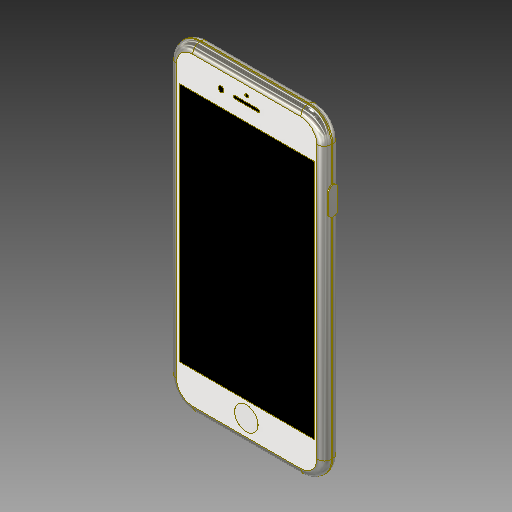
# Autodesk Inventor part: Iphone - Athena H
Saved by Autodesk Inventor 2019 (Build 230136000, 136)
## iProperties
Created: 2018-11-30
Part Number: Iphone - Athena H
Material: Generic
Document SubType Name: Modeling
Designer: mhs
Density: 1 g/cm^3
Appearance: Default
Author: mhs
Autodesk Inventor part; units mm, degrees
ref_plane "YZ Plane" through (0, 0, 0) normal (1, 0, 0) x (0, 1, 0)
ref_plane "XZ Plane" through (0, 0, 0) normal (0, 1, 0) x (-1, 0, 0)
ref_plane "XY Plane" through (0, 0, 0) normal (0, 0, 1) x (1, 0, 0)
sketch "Sketch1" plane through (0, 0, 0) normal (0, 0, 1) x (1, 0, 0)
  line L0 (10.16, 0) -> (56.896, 0)
  line L1 (67.056, 10.16) -> (67.056, 128.016)
  line L2 (56.896, 138.176) -> (10.16, 138.176)
  line L3 (0, 128.016) -> (0, 10.16)
  arc A0 (10.16, 138.176) -> (0, 128.016) centre (10.16, 128.016) ccw
  arc A1 (67.056, 128.016) -> (56.896, 138.176) centre (56.896, 128.016) ccw
  arc A2 (56.896, 0) -> (67.056, 10.16) centre (56.896, 10.16) ccw
  arc A3 (0, 10.16) -> (10.16, 0) centre (10.16, 10.16) ccw
  line L4 (4.318, 121.158) -> (62.738, 121.158)
  line L5 (62.738, 121.158) -> (62.738, 17.018)
  line L6 (62.738, 17.018) -> (4.318, 17.018)
  line L7 (4.318, 17.018) -> (4.318, 121.158)
  point P0 (0, 0)
  point P1 (67.056, 138.176)
  point P2 (67.056, 0)
  point P3 (0, 138.176)
  dimension "d0" = 67.056
  dimension "d1" = 138.176
  dimension "d2" = 10.16
  dimension "d3" = 58.42
  dimension "d4" = 104.14
  dimension "d5" = 17.018
  dimension "d6" = 4.318
  constraints: 16 end point, 8 point on circle, 8 point on line, 8 tangent, 4 centre point, 4 parallel, 3 equal radius, 2 horizontal, 2 perpendicular
  measures "d0" distance of point (67.056, 138.176) point (0, 138.176)
  measures "d1" distance of point (67.056, 0) point (67.056, 138.176)
  measures "d2" radius of A0
  measures "d3" distance of L4.start L4.end
  measures "d4" distance of L4.end L5.end
  measures "d5" distance between parallel lines of L0 L6
  measures "d6" distance between parallel lines of L3 L7
extrude "Extrusion1" add sketch "Sketch1" along normal blind 6.858 contours A3 L3 A0 L2 A1 L1 A2 L0 | L4 L5 L6 L7
fillet "Fillet1" radius 3.175 16 edges at (64.0802, 135.2002, 6.858) (33.528, 138.176, 6.858) (2.9758, 135.2002, 6.858) (0, 69.088, 6.858) (2.9758, 2.9758, 6.858) (33.528, 0, 6.858) (64.0802, 2.9758, 6.858) (67.056, 69.088, 6.858) (64.0802, 135.2002, 0) (33.528, 138.176, 0) (2.9758, 135.2002, 0) (0, 69.088, 0) (2.9758, 2.9758, 0) (33.528, 0, 0) (64.0802, 2.9758, 0) (67.056, 69.088, 0)
sketch "Sketch2" plane through (0, 0, 6.858) normal (0, 0, 1) x (1, 0, 0)
  line L0 (4.318, 121.158) -> (62.738, 121.158)
  line L1 (62.738, 121.158) -> (62.738, 17.018)
  line L2 (62.738, 17.018) -> (4.318, 17.018)
  line L3 (4.318, 17.018) -> (4.318, 121.158)
  line L4 (56.896, 138.176) -> (10.16, 138.176) projected
  line L5 (0, 128.016) -> (0, 10.16) projected
  point P0 (0, 0)
  dimension "d10" = 104.14
  dimension "d11" = 58.42
  dimension "d12" = 17.018
  dimension "d13" = 4.318
  constraints: 8 end point, 2 parallel, 1 horizontal, 1 perpendicular
  measures "d10" distance of L2.end L0.start
  measures "d11" distance of L0.start L0.end
  measures "d12" distance between parallel lines of L4 L0
  measures "d13" distance between parallel lines of L3 L5
extrude "Extrusion2" add sketch "Sketch2" along normal blind 0.0254
sketch "Sketch3" plane through (0, 0, 6.858) normal (0, 0, 1) x (1, 0, 0)
  circle A0 centre (33.401, 10.3132) radius 5.08
  line L0 (63.881, 128.016) -> (63.881, 10.16) projected
  point P0 (0, 0)
  dimension "d16" = 10.16
  dimension "d17" = 30.48
  constraints: 1 centre point
  measures "d16" diameter of A0
  measures "d17" distance from line of L0 A0.centre
extrude "Extrusion3" add sketch "Sketch3" along normal blind 0.0254
sketch "Sketch4" plane through (0, 0, 6.858) normal (0, 0, 1) x (1, 0, 0)
  line L0 (28.448, 128.016) -> (38.608, 128.016) construction
  line L1 (10.16, 135.001) -> (56.896, 135.001) projected
  line L2 (28.448, 127.381) -> (38.608, 127.381)
  line L3 (38.608, 128.651) -> (28.448, 128.651)
  arc A0 (28.448, 128.651) -> (28.448, 127.381) centre (28.448, 128.016) ccw
  arc A1 (38.608, 127.381) -> (38.608, 128.651) centre (38.608, 128.016) ccw
  circle A2 centre (22.479, 128.016) radius 1.27
  circle A3 centre (33.528, 131.1287) radius 0.762
  point P0 (0, 0)
  point P1 (33.528, 128.016)
  point P2 (33.528, 135.001)
  point P3 (33.528, 128.651)
  point P4 (63.881, 128.016)
  point P5 (39.243, 128.016)
  point P6 (3.175, 128.016)
  dimension "d20" = 1.27
  dimension "d21" = 10.16
  dimension "d22" = 2.54
  dimension "d23" = 4.064
  dimension "d24" = 1.524
  dimension "d25" = 2.4777
  constraints: 8 end point, 5 point on circle, 4 centre point, 4 tangent, 3 midpoint, 2 horizontal alignment, 2 parallel, 1 vertical alignment
  measures "d20" diameter of A1
  measures "d21" distance of L2.start L2.end
  measures "d22" diameter of A2
  measures "d24" diameter of A3
  measures "d25" distance from line of A3.centre L3
extrude "Extrusion4" cut sketch "Sketch4" against normal blind 0.0254
sketch "Sketch5" plane through (0, 0, 0) normal (0, 0, -1) x (-1, 0, 0)
  circle A0 centre (-52.7685, 127.0635) radius 3.175
  line L0 (-63.881, 10.16) -> (-63.881, 128.016) projected
  line L1 (-56.896, 135.001) -> (-10.16, 135.001) projected
  point P0 (0, 0)
  dimension "d28" = 6.35
  dimension "d29" = 11.1125
  dimension "d30" = 4.7625
  constraints: 1 centre point
  measures "d28" diameter of A0
  measures "d29" distance from line of A0.centre L0
  measures "d30" distance edge to line of A0 L1
extrude "Extrusion5" add sketch "Sketch5" along normal blind 1.27 draft -10
sketch "Sketch6" plane through (0, 0, 0) normal (0, 0, -1) x (-1, 0, 0)
  circle A0 centre (-46.4185, 127.0635) radius 0.5
  circle A1 centre (-40.0685, 127.0635) radius 2
  line L0 (-56.896, 135.001) -> (-10.16, 135.001) projected
  circle A2 centre (-52.7685, 127.0635) radius 2.9511 projected
  point P0 (0, 0)
  dimension "d33" = 1
  dimension "d34" = 4
  dimension "d35" = 7.9375
  dimension "d36" = 7.9375
  dimension "d37" = 6.35
  dimension "d38" = 6.35
  constraints: 2 centre point
  measures "d33" diameter of A0
  measures "d34" diameter of A1
  measures "d35" distance from line of L0 A1.centre
  measures "d36" distance from line of L0 A0.centre
  measures "d37" distance of A0.centre A2.centre
  measures "d38" distance of A0.centre A1.centre
extrude "Extrusion6" add sketch "Sketch6" along normal blind 0.0254 contours A0 | A1
sketch "Sketch7" plane through (67.056, 10.16, 3.175) normal (1, 0, 0) x (0, 0, -1)
  line L0 (-0.254, 100.856) -> (-0.254, 92.856) construction
  line L1 (0, 117.856) -> (0, 0) projected
  line L2 (-2.254, 100.856) -> (-2.254, 92.856)
  line L3 (1.746, 92.856) -> (1.746, 100.856)
  arc A0 (1.746, 100.856) -> (-2.254, 100.856) centre (-0.254, 100.856) ccw
  arc A1 (-2.254, 92.856) -> (1.746, 92.856) centre (-0.254, 92.856) ccw
  line L4 (0, 117.856) -> (-0.508, 117.856) projected
  line L5 (3.175, 117.856) -> (0, 117.856) projected
  point P0 (3.175, -10.16)
  point P1 (-0.254, 96.856)
  point P2 (-0.254, 117.856)
  dimension "d41" = 8
  dimension "d42" = 2
  dimension "d43" = 17
  constraints: 8 end point, 4 point on circle, 4 tangent, 2 centre point, 2 midpoint, 2 parallel, 1 vertical alignment
  measures "d41" distance of L2.start L2.end
  measures "d42" radius of A0
  measures "d43" distance from line of L0.start L5
extrude "Extrusion7" add sketch "Sketch7" along normal blind 0.508
sketch "Sketch8" plane through (0, 10.16, 3.175) normal (-1, 0, 0) x (0, 0, 1)
  line L0 (0.254, 113.856) -> (0.254, 109.856) construction
  line L1 (0, 117.856) -> (0, 102.8398) projected
  line L2 (-1.246, 113.856) -> (-1.246, 109.856)
  line L3 (1.754, 109.856) -> (1.754, 113.856)
  arc A0 (1.754, 113.856) -> (-1.246, 113.856) centre (0.254, 113.856) ccw
  arc A1 (-1.246, 109.856) -> (1.754, 109.856) centre (0.254, 109.856) ccw
  line L4 (0.254, 101.856) -> (0.254, 81.856) construction
  line L5 (-1.746, 101.856) -> (-1.746, 81.856)
  line L6 (2.254, 81.856) -> (2.254, 101.856)
  arc A2 (2.254, 101.856) -> (-1.746, 101.856) centre (0.254, 101.856) ccw
  arc A3 (-1.746, 81.856) -> (2.254, 81.856) centre (0.254, 81.856) ccw
  line L7 (0, 117.856) -> (0.508, 117.856) projected
  point P0 (-3.175, -10.16)
  point P1 (0.254, 111.856)
  point P2 (0.254, 91.856)
  point P3 (0.254, 117.856)
  point P4 (0.254, 117.856)
  dimension "d46" = 1.5
  dimension "d47" = 2
  dimension "d48" = 4
  dimension "d49" = 4
  dimension "d50" = 8
  dimension "d51" = 20
  constraints: 16 end point, 8 point on circle, 8 tangent, 4 centre point, 4 midpoint, 3 parallel, 2 point on line, 2 vertical alignment
  measures "d46" radius of A0
  measures "d47" radius of A2
  measures "d48" distance of L3.start L3.end
  measures "d49" distance of point (0.254, 117.856) L0.start
  measures "d50" distance of L4.start L0.end
  measures "d51" distance of L6.start L6.end
extrude "Extrusion8" cut sketch "Sketch8" against normal blind 0.254
sketch "Sketch9" plane through (0.254, 10.16, 3.175) normal (-1, 0, 0) x (0, 0, 1)
  line L0 (-0.2303, 114.356) -> (-0.2303, 109.356) construction
  line L1 (0, 117.856) -> (0, 102.8398) projected
  line L2 (-0.9803, 114.356) -> (-0.9803, 109.356)
  line L3 (0.5197, 109.356) -> (0.5197, 114.356)
  arc A0 (0.5197, 114.356) -> (-0.9803, 114.356) centre (-0.2303, 114.356) ccw
  arc A1 (-0.9803, 109.356) -> (0.5197, 109.356) centre (-0.2303, 109.356) ccw
  arc A2 (1.7523, 113.9265) -> (-1.2443, 113.9265) centre (0.254, 113.856) ccw projected
  line L4 (-1.2443, 109.7855) -> (-1.2443, 113.9265) projected
  line L5 (0.2015, 101.856) -> (0.2015, 95.2367) construction
  line L6 (0, 102.8398) -> (0, 90.8722) projected
  line L7 (-0.9657, 101.856) -> (-0.9657, 95.2367)
  line L8 (1.3686, 95.2367) -> (1.3686, 101.856)
  arc A3 (1.3686, 101.856) -> (-0.9657, 101.856) centre (0.2015, 101.856) ccw
  arc A4 (-0.9657, 95.2367) -> (1.3686, 95.2367) centre (0.2015, 95.2367) ccw
  line L9 (0.2015, 81.6901) -> (0.2015, 88.3094) construction
  line L10 (0, 90.8722) -> (0, 0) projected
  line L11 (-0.9657, 81.6901) -> (-0.9657, 88.3094)
  line L12 (1.3686, 88.3094) -> (1.3686, 81.6901)
  arc A5 (-0.9657, 81.6901) -> (1.3686, 81.6901) centre (0.2015, 81.6901) ccw
  arc A6 (1.3686, 88.3094) -> (-0.9657, 88.3094) centre (0.2015, 88.3094) ccw
  arc A7 (1.7523, 103.1808) -> (-1.2443, 103.1808) centre (0.254, 101.856) ccw projected
  point P0 (-3.175, -10.16)
  point P1 (-0.2303, 111.856)
  point P2 (-1.2443, 111.856)
  point P3 (0.2015, 98.5463)
  point P4 (0.2015, 84.9998)
  dimension "d54" = 0.75
  dimension "d55" = 5
  dimension "d58" = 0
  constraints: 24 end point, 12 point on circle, 12 tangent, 6 centre point, 6 parallel, 4 midpoint, 1 collinear, 1 equal radius, 1 horizontal alignment
  measures "d54" radius of A1
  measures "d55" distance of L2.start L2.end
  measures "d58" vertical distance of L5.start A7.centre
extrude "Extrusion9" add sketch "Sketch9" along normal blind 0.762
sketch "Sketch10" plane through (10.16, 0, 3.175) normal (0, -1, 0) x (1, 0, 0)
  line L0 (19.6718, 0.254) -> (27.0642, 0.254) construction
  line L1 (0, 0) -> (46.736, 0) projected
  line L2 (19.6718, 1.3655) -> (27.0642, 1.3655)
  line L3 (27.0642, -0.8575) -> (19.6718, -0.8575)
  arc A0 (19.6718, 1.3655) -> (19.6718, -0.8575) centre (19.6718, 0.254) ccw
  arc A1 (27.0642, -0.8575) -> (27.0642, 1.3655) centre (27.0642, 0.254) ccw
  line L4 (0, 0.508) -> (46.736, 0.508) projected
  circle A2 centre (3.0836, 0.254) radius 1.0799
  circle A3 centre (5.9129, 0.254) radius 0.5147
  circle A4 centre (34.9269, 0.254) radius 0.5147
  circle A5 centre (36.2103, 0.254) radius 0.5147
  circle A6 centre (37.4937, 0.254) radius 0.5147
  circle A7 centre (38.7772, 0.254) radius 0.5147
  circle A8 centre (40.0606, 0.254) radius 0.5147
  circle A9 centre (41.344, 0.254) radius 0.5147
  point P0 (-10.16, -3.175)
  point P1 (23.368, 0.254)
  point P2 (23.368, 0.508)
  dimension "d61" = 7.3925
  dimension "d62" = 0.254
  dimension "d63" = 0.254
  dimension "d64" = 0.254
  dimension "d65" = 0.254
  dimension "d66" = 0.254
  dimension "d67" = 0.254
  constraints: 10 centre point, 8 end point, 6 equal radius, 4 point on circle, 4 tangent, 2 midpoint, 2 parallel, 1 vertical alignment
  measures "d61" distance of L3.start L3.end
  measures "d62" distance from line of L1 point (23.368, 0.254)
extrude "Extrusion10" cut sketch "Sketch10" against normal blind 17.78 contours A2 L4 L1 | L1 A2 | A2 L4 | A3 L4 L1 | L1 A3 | A3 L4 | A0 L4 A1 L1 | L1 A1 L3 A0 | A0 L2 A1 L4 | A4 L4 L1 | L1 A4 | A4 L4 | A5 L4 L1 | L1 A5 | A5 L4 | A6 L4 L1 | L1 A6 | A6 L4 | A7 L4 L1 | L1 A7 | A7 L4 | A8 L4 L1 | L1 A8 | A8 L4 | A9 L4 L1 | L1 A9 | A9 L4
body "Solid1"
